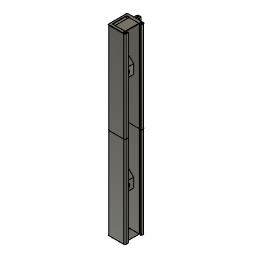
Rainbow_Matchstick_Mount (Autodesk Fusion 360 design; units mm, degrees)
Autodesk Fusion 360 part; units mm, degrees
sketch "Base" plane through (0, 0, 0) normal (0, 0, 1) x (1, 0, 0) in component "Clip"
  line L0 (0, 0) -> (15, 0)
  line L1 (15, 0) -> (15, -3)
  line L2 (15, -3) -> (14, -3)
  line L3 (14, -3) -> (14, -1)
  line L4 (14, -1) -> (13, -1)
  line L5 (13, -16) -> (14, -16)
  line L6 (14, -16) -> (14, -14)
  line L7 (14, -14) -> (15, -14)
  line L8 (15, -14) -> (15, -17)
  line L9 (15, -17) -> (0, -17)
  line L10 (0, -17) -> (0, 0)
  line L11 (13, -1) -> (13, -2.5)
  line L12 (13, -2.5) -> (8, -2.5)
  line L13 (8, -2.5) -> (8, -14.5)
  line L14 (8, -14.5) -> (13, -14.5)
  line L15 (13, -14.5) -> (13, -16)
  line L16 (6, 0) -> (6, 0.45)
  line L17 (6, 0.45) -> (5.7, 1.25)
  line L18 (5.7, 1.25) -> (6.4, 3.25)
  line L19 (6.4, 3.25) -> (7.1, 3.25)
  line L20 (7.1, 3.25) -> (7.1, 0)
  line L21 (7.9, 0) -> (7.9, 3.25)
  line L22 (7.9, 3.25) -> (8.6, 3.25)
  line L23 (8.6, 3.25) -> (9.3, 1.25)
  line L24 (9.3, 1.25) -> (9, 0.45)
  line L25 (9, 0.45) -> (9, 0)
  line L26 (5.7, 1.25) -> (7.1, 1.25) construction
  line L27 (9.3, 1.25) -> (7.9, 1.25) construction
  line L28 (7.9, 160.3492) -> (9, 160.3492) construction
  line L29 (6, 46112.2109) -> (7.1, 46112.2109) construction
  line L30 (7.9, 74203.3535) -> (9, 74203.3535) construction
  line L31 (7.1, 322921.7824) -> (7.9, 322921.7824) construction
  line L32 (7.5, 322921.7824) -> (7.5, 0) construction
  line L33 (8, -8.5) -> (0, -8.5) construction
  dimension "d3" = 12
  dimension "d7" = 17
  dimension "d8" = 8
  dimension "diffuser_height" = 15
  dimension "d10" = 1
  dimension "d12" = 1
  dimension "diffuser_thickness" = 1
  dimension "d14" = 5
  dimension "d15" = 15
  dimension "d18" = 0.7
  dimension "snap_length" = 2.8
  dimension "snap_outer" = 3.6
  dimension "d22" = 0.8
  dimension "snap_inner" = 3
  dimension "d26" = 0.8
  dimension "d42" = 2
  dimension "snap_base" = 0.45
  dimension "d91" = 3
  constraint coincident L0.start L10.end
  constraint horizontal L0
  constraint perpendicular L0 L1
  constraint perpendicular L1 L2
  constraint perpendicular L2 L3
  constraint perpendicular L3 L4
  constraint perpendicular L5 L6
  constraint perpendicular L6 L7
  constraint perpendicular L7 L8
  constraint perpendicular L8 L9
  constraint perpendicular L0 L10
  constraint equal L4 L5
  constraint equal L2 L7
  constraint perpendicular L4 L11
  constraint perpendicular L11 L12
  constraint perpendicular L4 L13
  constraint perpendicular L13 L14
  constraint perpendicular L5 L15
  constraint collinear L1 L8
  constraint equal L11 L15
  constraint equal L1 L8
  constraint coincident L9.end L10.start
  constraint coincident L0 L16.start
  constraint perpendicular L0 L16
  constraint perpendicular L16 L19
  constraint coincident L0 L20.end
  constraint perpendicular L0 L20
  constraint coincident L0 L21.start
  constraint perpendicular L0 L21
  constraint perpendicular L21 L22
  constraint coincident L0 L25.end
  constraint perpendicular L0 L25
  constraint equal L19 L22
  constraint coincident L20 L26.end
  constraint perpendicular L20 L26
  constraint coincident L21 L27.end
  constraint perpendicular L21 L27
  constraint equal L26 L27
  constraint collinear L19 L22
  constraint collinear L26 L27
  constraint coincident L21 L28.start
  constraint perpendicular L25 L28
  constraint coincident L25 L28.end
  constraint equal L17 L24
  constraint coincident L16 L29.start
  constraint coincident L20 L29.end
  constraint perpendicular L20 L29
  constraint coincident L21 L30.start
  constraint coincident L25 L30.end
  constraint perpendicular L25 L30
  constraint equal L29 L30
  constraint coincident L20 L31.start
  constraint coincident L21 L31.end
  constraint perpendicular L21 L31
  constraint midpoint L31 L32.start
  constraint coincident L0 L32.end
  constraint perpendicular L0 L32
  constraint midpoint L0 L32.end
  constraint midpoint L13 L33.start
  constraint midpoint L10 L33.end
  constraint perpendicular L10 L33
  measures "d3" distance of L12.end L13.end
  measures "d7" distance of L0 L9
  measures "d8" distance of L10 L13
  measures "diffuser_height" distance of L4 L5
  measures "d10" distance of L5 L9
  measures "d12" distance of L6.end L7.end
  measures "diffuser_thickness" distance of L5.start L5.end
  measures "d14" distance of L13.end L14.end
  measures "d15" distance of L8.end L9.end
  measures "d18" distance of L18.end L19.end
  measures "snap_length" vertical distance of L22.end L24.end
  measures "snap_outer" distance of L17.end L23.end
  measures "d22" distance of L20 L21
  measures "snap_inner" distance of L16 L25
  measures "d26" distance of L16.end L26
  measures "d42" distance of L19 L26
  measures "snap_base" distance of L24.end L25.end
  measures "d91" distance of L0.end L1.end
extrude "Extrude1" add sketch "Base" along normal blind 158 contours L0 L1 L2 L3 L4 L5 L6 L7 L8 L9 L10 L11 L12 L13 L14 L15 makes body 1 in component "Clip"
sketch "Sketch1" plane through (8, 0, 0) normal (1, 0, 0) x (0, 1, 0) in component "PCB"
  line L0 (-14.5, 0) -> (-2.5, 0)
  line L1 (-2.5, 0) -> (-2.5, 158)
  line L2 (-2.5, 158) -> (-14.5, 158)
  line L3 (-14.5, 158) -> (-14.5, 0)
  line L4 (-8.5, 158) -> (-8.5, 121.2) construction
  line L5 (-8.5, 0) -> (-8.5, 36.15) construction
  circle A0 centre (-8.5, 121.2) radius 1.6
  circle A1 centre (-8.5, 36.15) radius 1.6
  dimension "d75" = 36.8
  dimension "d76" = 36.15
  dimension "d77" = 3.2
  dimension "d78" = 3.2
  constraint midpoint L2 L4.start
  constraint perpendicular L2 L4
  constraint midpoint L0 L5.start
  constraint perpendicular L0 L5
  constraint coincident L4.end A0.centre
  constraint coincident L5.end A1.centre
  measures "d75" distance of L4.start L4.end
  measures "d76" distance of L5.start L5.end
  measures "d77" diameter of A0
  measures "d78" diameter of A1
extrude "Extrude1'" add sketch "Sketch1" along normal blind 1.57 separate body makes body 2 in component "PCB"
chamfer "Chamfer1" distance 2.8 distance2 4 2 edges at (8.785, -14.5, 158) (8.785, -2.5, 0) measured on face at (8.5233, -6.5, 158) measured on face at (8.5233, -10.5, 0) on bodies 2 in component "PCB"
chamfer "Chamfer1" distance 4 distance2 2.8 2 edges at (8.785, -2.5, 158) (8.785, -14.5, 0) measured on face at (9.0467, -2.5, 52.6667) measured on face at (9.0467, -14.5, 105.3333) on bodies 2 in component "PCB"
sketch "Holes" plane through (8, 0, 0) normal (1, 0, 0) x (0, 1, 0) in component "Clip"
  line L0 (-14.5, 0) -> (-2.5, 0)
  line L1 (-2.5, 0) -> (-2.5, 158)
  line L2 (-2.5, 158) -> (-14.5, 158)
  line L3 (-14.5, 158) -> (-14.5, 0)
  circle A0 centre (-8.5, 36.15) radius 2.35
  line L4 (-8.5, 36.15) -> (-8.5, 46.15) construction
  line L5 (-8.5, 36.15) -> (-8.5, 26.15) construction
  line L6 (-14.5, 46.15) -> (-2.5, 46.15)
  line L7 (-14.5, 26.15) -> (-2.5, 26.15)
  circle A1 centre (-8.5, 36.15) radius 1.6
  circle A2 centre (-8.5, 121.2) radius 1.6 construction
  circle A3 centre (-8.5, 121.2) radius 2.35
  line L8 (-8.5, 121.2) -> (-8.5, 131.2) construction
  line L9 (-8.5, 121.2) -> (-8.5, 111.2) construction
  line L10 (-14.5, 131.2) -> (-2.5, 131.2)
  line L11 (-2.5, 111.2) -> (-14.5, 111.2)
  dimension "d45" = 4.7
  dimension "d70" = 10
  dimension "d85" = 4.7
  dimension "d86" = 10
  constraint concentric A0 A1
  constraint coincident A0.centre L4.start
  constraint vertical L4
  constraint parallel L4 L5
  constraint coincident L3 L6.start
  constraint coincident L1 L6.end
  constraint perpendicular L1 L6
  constraint coincident L4.end L6
  constraint coincident L3 L7.start
  constraint coincident L1 L7.end
  constraint perpendicular L1 L7
  constraint coincident L5.end L7
  constraint equal L4 L5
  constraint concentric A2 A3
  constraint coincident A2.centre A3.centre
  constraint vertical L8
  constraint parallel L8 L9
  constraint equal L8 L9
  constraint coincident L3 L10.start
  constraint coincident L1 L10.end
  constraint perpendicular L1 L10
  constraint coincident L1 L11.start
  constraint coincident L3 L11.end
  constraint perpendicular L3 L11
  constraint coincident L9.end L11
  constraint coincident L8.end L10
  measures "d45" diameter of A0
  measures "d70" distance of A0.centre L4.end
  measures "d85" diameter of A3
  measures "d86" distance of A2.centre L8.end
extrude "Extrude2" cut sketch "Holes" against normal blind 4 contours A0 | A1 | A3 bodies 1 in component "Clip"
extrude "Extrude9" cut sketch "Holes" against normal blind 6 contours L0 L1 L3 L7 | L1 L3 L6 L11 | L1 L2 L3 L10 | A3 bodies 1 in component "Clip"
chamfer "Chamfer5" distance 6 angle 45 4 edges at (8, -8.5, 46.15) (8, -8.5, 26.15) (8, -8.5, 111.2) (8, -8.5, 131.2) on bodies 1 in component "Clip"
sketch "Sketch3" plane through (0, 0, 0) normal (0, 0, -1) x (1, 0, 0) in component "Clip"
  line L0 (2, 14.5) -> (13, 14.5)
  line L1 (13, 14.5) -> (13, 16)
  line L2 (13, 16) -> (14, 16)
  line L3 (14, 16) -> (14, 14)
  line L4 (14, 14) -> (15, 14)
  line L5 (15, 14) -> (15, 17)
  line L6 (15, 17) -> (0, 17)
  line L7 (0, 17) -> (0, 0)
  line L8 (0, 0) -> (15, 0)
  line L9 (15, 0) -> (15, 3)
  line L10 (15, 3) -> (14, 3)
  line L11 (14, 3) -> (14, 1)
  line L12 (14, 1) -> (13, 1)
  line L13 (13, 1) -> (13, 2.5)
  line L14 (13, 2.5) -> (2, 2.5)
  line L15 (2, 2.5) -> (2, 14.5)
  line L16 (13, 14.5) -> (13, 2.5)
  line L17 (4, 2.5) -> (4, 14.5)
  dimension "d97" = 2
  constraint coincident L0.end L1.start
  constraint coincident L13.end L14.start
  constraint coincident L14 L17.start
  constraint coincident L0 L17.end
  constraint perpendicular L0 L17
  measures "d97" distance of L15 L17
extrude "Extrude13" add sketch "Sketch3" against normal blind 0.2 contours L0 L14 L16 L17 bodies 1 in component "Clip"
extrude "Extrude14" add sketch "Sketch3" along normal blind 0.2 from surface at -158 contours L0 L14 L16 L17 bodies 1 in component "Clip"
extrude "Extrude7" add sketch "Base" along normal blind 10 contours L0 L16 L17 L18 L19 L20 | L0 L21 L22 L23 L24 L25 bodies 1 in component "Clip"
extrude "Extrude8" add sketch "Base" against normal blind 10 from surface at 158 contours L0 L16 L17 L18 L19 L20 | L0 L21 L22 L23 L24 L25 bodies 1 in component "Clip"
extrude "Extrude10" add sketch "Base" along normal mid plane 20 from surface at 79 contours L0 L16 L17 L18 L19 L20 | L0 L21 L22 L23 L24 L25 bodies 1 in component "Clip"
chamfer "Chamfer4" distance 3.25 angle 45 8 edges at (8.25, 3.25, 148) (6.75, 3.25, 148) (8.25, 3.25, 10) (6.75, 3.25, 10) (6.75, 3.25, 69) (8.25, 3.25, 69) (6.75, 3.25, 89) (8.25, 3.25, 89) on bodies 1 in component "Clip"
fillet "Fillet1" radius 1 4 edges at (0, -17, 79) (15, -17, 79) (0, 0, 79) (15, 0, 79) on bodies 1 in component "Clip"
chamfer "Chamfer6" distance 0.2 distance2 0.2 44 edges at (3.5, 0, 158) (0.2929, -0.2929, 158) (0, -8.5, 158) (0.2929, -16.7071, 158) (7.5, -17, 158) (14.7071, -16.7071, 158) (15, -15, 158) (11.5, 0, 158) (15, -2, 158) (14.7071, -0.2929, 158) (7.5, 0, 158) (14.5, -3, 158) (14, -2, 158) (13.5, -1, 158) (13, -8.5, 158) (13.5, -16, 158) (14, -15, 158) (14.5, -14, 158) (4, -8.5, 158) (3, -2.5, 158) (2, -8.5, 158) (3, -14.5, 158) (13, -8.5, 0) (13.5, -16, 0) (14, -15, 0) (14.5, -14, 0) (15, -15, 0) (14.7071, -16.7071, 0) (7.5, -17, 0) (0.2929, -16.7071, 0) (0, -8.5, 0) (0.2929, -0.2929, 0) (3.5, 0, 0) (2, -8.5, 0) (3, -14.5, 0) (4, -8.5, 0) (3, -2.5, 0) (7.5, 0, 0) (11.5, 0, 0) (14.7071, -0.2929, 0) (15, -2, 0) (14.5, -3, 0) (14, -2, 0) (13.5, -1, 0) measured on face at (7, -11, 158) measured on face at (0.5, -0.134, 52.6667) measured on face at (7, -11, 158) measured on face at (0.134, -16.5, 52.6667) measured on face at (7, -11, 158) measured on face at (14.6691, -16.7431, 52.6667) measured on face at (7, -11, 158) measured on face at (7, -11, 158) measured on face at (7, -11, 158) measured on face at (14.5, -0.134, 52.6667) measured on face at (7, -11, 158) measured on face at (7, -11, 158) measured on face at (7, -11, 158) measured on face at (7, -11, 158) measured on face at (7, -11, 158) measured on face at (7, -11, 158) measured on face at (7, -11, 158) measured on face at (7, -11, 158) measured on face at (4, -6.5, 157.9333) measured on face at (7, -11, 158) measured on face at (7, -11, 158) measured on face at (7, -11, 158) measured on face at (7, -11, 0) measured on face at (7, -11, 0) measured on face at (7, -11, 0) measured on face at (7, -11, 0) measured on face at (7, -11, 0) measured on face at (14.6691, -16.7431, 52.6667) measured on face at (7, -11, 0) measured on face at (0.134, -16.5, 52.6667) measured on face at (7, -11, 0) measured on face at (0.5, -0.134, 52.6667) measured on face at (7, -11, 0) measured on face at (7, -11, 0) measured on face at (7, -11, 0) measured on face at (4, -6.5, 0.0667) measured on face at (7, -11, 0) measured on face at (7, -11, 0) measured on face at (7, -11, 0) measured on face at (14.5, -0.134, 52.6667) measured on face at (7, -11, 0) measured on face at (7, -11, 0) measured on face at (7, -11, 0) measured on face at (7, -11, 0) on bodies 1 in component "Clip"
chamfer "Chamfer3" distance 0.2 angle 45 2 edges at (8, -10.691, 36.9998) (8, -10.691, 122.0498) on bodies 1 in component "Clip"
ref_plane "WorkPlane1" through (0, 0, 79) normal (0, 0, 1) x (1, 0, 0) in component "Clip"
split "Split1" by plane through (0, 0, 79) normal (0, 0, 1) bodies 1 makes body 3 at (0, -11, 105.2667) in component "Clip"
component "Clip" placed x (1, 0, 0) y (0, 1, 0) z (0, 0, 1) at (0, 0, 0)
component "PCB" placed x (1, 0, 0) y (0, 1, 0) z (0, 0, 1) at (0, 0, 0)
equation "snap_height = 10 mm"
equation "d67 = -snap_height"
equation "d69 = snap_length + snap_base"
equation "d88 = snap_height"
named bodies: "Left_Back", "Left_Front"
